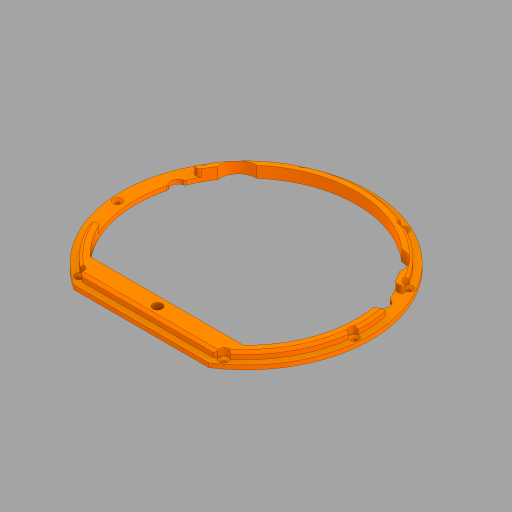
# Autodesk Inventor part: ramka_kriska
Saved by Autodesk Inventor 2024.2 (Build 282272000, 272)
## iProperties
Created: 2024-01-02
Part Number: ramka_kriska
Material: Типовые
Document SubType Name: Modeling
Designer: Fedor Orlov
Density: 1 g/cm^3
Appearance: По умолчанию
Author: Fedor Orlov
Autodesk Inventor part; units mm, degrees
ref_plane "YZ Plane" through (0, 0, 0) normal (1, 0, 0) x (0, 1, 0)
ref_plane "XZ Plane" through (0, 0, 0) normal (0, 1, 0) x (-1, 0, 0)
ref_plane "XY Plane" through (0, 0, 0) normal (0, 0, 1) x (1, 0, 0)
sketch "Эскиз2" plane through (0, 0, 0) normal (0, 1, 0) x (-1, 0, 0)
  circle A0 centre (52.9444, -65.7473) radius 1.5
  circle A1 centre (18.9444, -65.7473) radius 1.5
  circle A2 centre (-32.9359, 24.112) radius 1.5
  circle A3 centre (-15.9359, 53.5568) radius 1.5
  circle A4 centre (87.8247, 53.5568) radius 1.5
  circle A5 centre (104.8247, 24.112) radius 1.5
  arc A6 (-9.0556, 75.9947) -> (-12.1486, 77.6696) centre (-11.0556, 75.9947) ccw construction
  arc A7 (-12.1486, 77.6696) -> (84.0374, 77.6696) centre (35.9444, 3.9738) ccw
  arc A8 (84.0374, 77.6696) -> (80.9444, 75.9947) centre (82.9444, 75.9947) ccw construction
  line L0 (80.9444, 75.9947) -> (80.9444, 72.0979) construction
  arc A9 (78.9444, 70.0979) -> (80.9444, 72.0979) centre (78.9444, 72.0979) ccw construction
  line L1 (78.9444, 70.0979) -> (-7.0556, 70.0979) construction
  arc A10 (-9.0556, 72.0979) -> (-7.0556, 70.0979) centre (-7.0556, 72.0979) ccw construction
  line L2 (-9.0556, 72.0979) -> (-9.0556, 75.9947) construction
  arc A11 (80.2513, 70.5839) -> (-9.0556, 70.1176) centre (35.9444, 3.9738) ccw construction
  line L3 (35.9444, 3.9738) -> (-51.7207, 11.6435) construction
  line L4 (-51.7207, 11.6435) -> (-47.7359, 11.2949) construction
  circle A12 centre (-47.7359, 11.2949) radius 1.5
  line L5 (35.9444, 3.9738) -> (-17.5291, 73.8636) construction
  circle A13 centre (-15.0984, 70.6868) radius 1.5
  line L6 (35.9444, 3.9738) -> (-1.246, -75.7813) construction
  line L7 (35.9444, 3.9738) -> (-40.2658, -40.0262) construction
  circle A14 centre (0.4445, -72.156) radius 1.5
  circle A15 centre (-36.8017, -38.0262) radius 1.5
  line L8 (35.9444, 3.9738) -> (35.9444, -84.0262) construction
  circle A16 centre (86.9873, 70.6868) radius 1.5
  circle A17 centre (119.6248, 11.2949) radius 1.5
  circle A18 centre (108.6906, -38.0262) radius 1.5
  circle A19 centre (71.4444, -72.156) radius 1.5
  line L9 (-7.0556, 70.0979) -> (78.9444, 70.0979) construction
  line L10 (35.9444, 70.0979) -> (35.9444, 66.5979) construction
  circle A20 centre (35.9444, 66.5979) radius 1.5
  line L11 (-19.0246, 62.0979) -> (90.9134, 62.0979)
  arc A21 (80.9444, 70.1176) -> (80.2513, 70.5839) centre (35.9444, 3.9738) ccw construction
  arc A22 (-9.0556, 70.1176) -> (-19.0246, 62.0979) centre (35.9444, 3.9738) ccw construction
  arc A23 (-19.0246, 62.0979) -> (90.9134, 62.0979) centre (35.9444, 3.9738) ccw
  arc A24 (90.9134, 62.0979) -> (80.9444, 70.1176) centre (35.9444, 3.9738) ccw construction
  arc A25 (-11.6466, 77.9947) -> (83.5354, 77.9947) centre (35.9444, 3.9738) ccw
  line L12 (83.5354, 77.9947) -> (-11.6466, 77.9947)
  arc A26 (83.5354, 77.9947) -> (-11.6466, 77.9947) centre (35.9444, 3.9738) ccw construction
  point P0 (0, 0)
  point P1 (60.9444, -70.7473)
  dimension "d30" = 8
  dimension "d55" = 95.182
  constraints: 34 point on circle, 27 centre point, 26 end point, 5 vertical, 4 coincident, 4 horizontal, 4 point on line, 4 symmetric about line, 1 midpoint, 72 other
  measures "d30" distance between parallel lines of L11 L1
  measures "d55" distance of L12.start L12.end
extrude "Выдавливание1" add sketch "Эскиз2" along normal blind 3 contours A25 L12 A7
fillet "Сопряжение1" radius 2 2 edges at (19.0246, 1.5, 62.0979) (-90.9134, 1.5, 62.0979)
sketch "Эскиз3" plane through (0, 3, 0) normal (0, 1, 0) x (1, 0, 0)
  arc A0 (11.6466, -77.9947) -> (-83.5354, -77.9947) centre (-35.9444, -3.9738) ccw projected
  circle A1 centre (-35.9444, -3.9738) radius 84
  arc A2 (11.6466, -77.9947) -> (-83.5354, -77.9947) centre (-35.9444, -3.9738) ccw projected
  line L0 (18.2228, -62.0979) -> (-90.1116, -62.0979) projected
  arc A3 (-91.5006, -61.537) -> (-90.1116, -62.0979) centre (-90.1116, -60.0979) ccw projected
  arc A4 (19.6117, -61.537) -> (-91.5006, -61.537) centre (-35.9444, -3.9738) ccw projected
  arc A5 (18.2228, -62.0979) -> (19.6117, -61.537) centre (18.2228, -60.0979) ccw projected
  circle A6 centre (-86.9873, -70.6868) radius 1.5 projected
  circle A7 centre (47.7359, -11.2949) radius 1.5 projected
  circle A8 centre (36.8017, 38.0262) radius 1.5 projected
  circle A9 centre (-0.4445, 72.156) radius 1.5 projected
  circle A10 centre (-108.6906, 38.0262) radius 1.5 projected
  circle A11 centre (-119.6248, -11.2949) radius 1.5 projected
  circle A12 centre (-71.4444, 72.156) radius 1.5 projected
  circle A13 centre (-35.9444, -66.5979) radius 1.5 projected
  circle A14 centre (15.0984, -70.6868) radius 1.5 projected
  line L1 (-83.5354, -77.9947) -> (11.6466, -77.9947) projected
  line L2 (-82.3456, -73.9947) -> (10.4568, -73.9947)
  point P0 (0, 0)
  point P1 (12.1486, -77.6696)
  point P2 (-84.0374, -77.6696)
  point P3 (-92.4829, -66.0979)
  point P4 (20.5941, -66.0979)
  point P5 (47.5919, -12.788)
  point P6 (47.8533, -9.7995)
  point P7 (37.5401, 36.7205)
  point P8 (36.0401, 39.3185)
  point P9 (0.9093, 71.51)
  point P10 (-1.8096, 72.7778)
  point P11 (-70.0793, 72.7778)
  point P12 (-72.7981, 71.51)
  point P13 (-107.929, 39.3185)
  point P14 (-109.4289, 36.7205)
  point P15 (-119.7422, -9.7995)
  point P16 (-119.4807, -12.788)
  point P17 (13.899, -71.5876)
  point P18 (16.2816, -69.7648)
  point P19 (-88.1704, -69.7648)
  point P20 (-85.7879, -71.5876)
  dimension "d34" = 4
  dimension "d56" = 4
  constraints: 4 point on circle, 2 end point, 1 centre point, 1 coincident, 1 horizontal
  measures "d34" radial gap between concentric circles of A0 A1
  measures "d56" distance between parallel lines of L2 L1
extrude "Выдавливание2" add sketch "Эскиз3" along normal blind 5 contours L2 A1 A6 A11 A10 A12 A9 A8 A7 A14
sketch "Эскиз4" plane through (0, 8, 0) normal (0, 1, 0) x (1, 0, 0)
  arc A0 (16.2816, -69.7648) -> (47.5919, -12.788) centre (-35.9444, -3.9738) ccw projected
  circle A1 centre (-35.9444, -66.5979) radius 1.5 projected
  arc A2 (18.2228, -62.0979) -> (19.6117, -61.537) centre (18.2228, -60.0979) ccw projected
  line L0 (18.2228, -62.0979) -> (-90.1116, -62.0979) projected
  arc A3 (-91.5006, -61.537) -> (-90.1116, -62.0979) centre (-90.1116, -60.0979) ccw projected
  arc A4 (19.6117, -61.537) -> (-91.5006, -61.537) centre (-35.9444, -3.9738) ccw projected
  arc A5 (-90.1116, -60.0979) -> (18.2228, -60.0979) centre (-35.9444, -3.9738) ccw construction
  line L1 (-90.1116, -60.0979) -> (18.2228, -60.0979)
  arc A6 (18.2228, -60.0979) -> (-90.1116, -60.0979) centre (-35.9444, -3.9738) ccw
  arc A7 (10.4568, -73.9947) -> (13.899, -71.5876) centre (-35.9444, -3.9738) ccw projected
  arc A8 (16.2816, -69.7648) -> (13.899, -71.5876) centre (15.0984, -70.6868) ccw projected
  arc A9 (47.8533, -9.7995) -> (47.5919, -12.788) centre (47.7359, -11.2949) ccw projected
  arc A10 (47.8533, -9.7995) -> (37.5401, 36.7205) centre (-35.9444, -3.9738) ccw projected
  arc A11 (36.0401, 39.3185) -> (37.5401, 36.7205) centre (36.8017, 38.0262) ccw projected
  arc A12 (36.0401, 39.3185) -> (0.9093, 71.51) centre (-35.9444, -3.9738) ccw projected
  arc A13 (-1.8096, 72.7778) -> (0.9093, 71.51) centre (-0.4445, 72.156) ccw projected
  arc A14 (-1.8096, 72.7778) -> (-70.0793, 72.7778) centre (-35.9444, -3.9738) ccw projected
  arc A15 (-72.7981, 71.51) -> (-70.0793, 72.7778) centre (-71.4444, 72.156) ccw projected
  arc A16 (-72.7981, 71.51) -> (-107.929, 39.3185) centre (-35.9444, -3.9738) ccw projected
  arc A17 (-109.4289, 36.7205) -> (-107.929, 39.3185) centre (-108.6906, 38.0262) ccw projected
  arc A18 (-109.4289, 36.7205) -> (-119.7422, -9.7995) centre (-35.9444, -3.9738) ccw projected
  arc A19 (-119.4807, -12.788) -> (-119.7422, -9.7995) centre (-119.6248, -11.2949) ccw projected
  arc A20 (-119.4807, -12.788) -> (-88.1704, -69.7648) centre (-35.9444, -3.9738) ccw projected
  arc A21 (-85.7879, -71.5876) -> (-88.1704, -69.7648) centre (-86.9873, -70.6868) ccw projected
  arc A22 (-85.7879, -71.5876) -> (-82.3456, -73.9947) centre (-35.9444, -3.9738) ccw projected
  line L2 (-82.3456, -73.9947) -> (10.4568, -73.9947) projected
  point P0 (0, 0)
  dimension "d38" = 2
  dimension "d39" = 2
  constraints: 4 point on circle, 2 centre point, 2 end point, 1 coincident, 1 horizontal
  measures "d38" radial gap between concentric circles of A4 A5
  measures "d39" distance between parallel lines of L0 L1
extrude "Выдавливание3" add sketch "Эскиз4" against normal blind 8 contours L0 A3 A4 A2
fillet "Сопряжение2" radius 2 2 edges at (18.2228, 4, 60.0979) (-90.1116, 4, 60.0979)
sketch "Эскиз5" plane through (0, 3, 0) normal (0, 1, 0) x (1, 0, 0)
  arc A0 (47.8533, -9.7995) -> (47.5919, -12.788) centre (47.7359, -11.2949) ccw projected
  arc A1 (36.0401, 39.3185) -> (37.5401, 36.7205) centre (36.8017, 38.0262) ccw projected
  arc A2 (-1.8096, 72.7778) -> (0.9093, 71.51) centre (-0.4445, 72.156) ccw projected
  arc A3 (-37.3586, -66.0979) -> (-34.5302, -66.0979) centre (-35.9444, -66.5979) ccw projected
  circle A4 centre (47.7359, -11.2949) radius 3.25
  circle A5 centre (36.8017, 38.0262) radius 3.25
  circle A6 centre (-0.4445, 72.156) radius 3.25
  circle A7 centre (-35.9444, -66.5979) radius 3.25
  circle A8 centre (-71.4444, 72.156) radius 1.5 projected
  circle A9 centre (-71.4444, 72.156) radius 3.25
  arc A10 (-109.4289, 36.7205) -> (-107.929, 39.3185) centre (-108.6906, 38.0262) ccw projected
  circle A11 centre (-108.6906, 38.0262) radius 3.25
  circle A12 centre (-119.6248, -11.2949) radius 1.5 projected
  circle A13 centre (-119.6248, -11.2949) radius 3.25
  circle A14 centre (15.0984, -70.6868) radius 1.5 projected
  circle A15 centre (15.0984, -70.6868) radius 3.25
  circle A16 centre (-86.9873, -70.6868) radius 1.5 projected
  circle A17 centre (-86.9873, -70.6868) radius 3.25
  point P0 (0, 0)
  dimension "d43" = 6.5
  dimension "d44" = 6.5
  dimension "d45" = 6.5
  dimension "d46" = 6.5
  dimension "d47" = 6.5
  dimension "d48" = 6.5
  dimension "d49" = 6.5
  dimension "d57" = 6.5
  dimension "d58" = 6.5
  constraints: 9 centre point, 9 coincident
  measures "d43" diameter of A4
  measures "d44" diameter of A5
  measures "d45" diameter of A6
  measures "d46" diameter of A7
  measures "d47" diameter of A9
  measures "d48" diameter of A11
  measures "d49" diameter of A13
  measures "d57" diameter of A15
  measures "d58" diameter of A17
extrude "Выдавливание4" cut sketch "Эскиз5" along normal blind 8 contours A4 | A5 | A6 | A7 | A8 | A9 | A11 | A12 | A13 | A14 | A15 | A16 | A17
chamfer "Фаска1" distance 1.6 angle 45 9 edges at (49.2359, 3, 11.2949) (38.3017, 3, -38.0262) (1.0555, 3, -72.156) (-69.9444, 3, -72.156) (-107.1906, 3, -38.0262) (-118.1248, 3, 11.2949) (-85.4873, 3, 70.6868) (16.5984, 3, 70.6868) (-34.4444, 3, 66.5979)
sketch "Эскиз6" plane through (0, 8, 0) normal (0, 1, 0) x (1, 0, 0)
  arc A0 (18.813, -59.5222) -> (-90.7019, -59.5222) centre (-35.9444, -3.9738) ccw projected
  arc A1 (9.3615, -73.9947) -> (10.2757, -73.3947) centre (-35.9444, -3.9738) ccw construction
  arc A2 (-74.3627, 70.7258) -> (-107.0114, 40.8088) centre (-35.9444, -3.9738) ccw projected
  line L0 (-82.1645, -73.3947) -> (10.2757, -73.3947)
  line L1 (-82.3456, -73.9947) -> (10.4568, -73.9947) projected
  arc A3 (47.9565, -8.0524) -> (47.3901, -14.5265) centre (47.7359, -11.2949) ccw projected
  arc A4 (47.9565, -8.0524) -> (38.372, 35.1807) centre (-35.9444, -3.9738) ccw projected
  arc A5 (35.1226, 40.8088) -> (38.372, 35.1807) centre (36.8017, 38.0262) ccw projected
  arc A6 (35.1226, 40.8088) -> (2.4739, 70.7258) centre (-35.9444, -3.9738) ccw projected
  arc A7 (-3.416, 73.4723) -> (2.4739, 70.7258) centre (-0.4445, 72.156) ccw projected
  arc A8 (-3.416, 73.4723) -> (-68.4728, 73.4723) centre (-35.9444, -3.9738) ccw projected
  arc A9 (-74.3627, 70.7258) -> (-68.4728, 73.4723) centre (-71.4444, 72.156) ccw projected
  arc A10 (-74.3627, 70.7258) -> (-107.0114, 40.8088) centre (-35.9444, -3.9738) ccw projected
  arc A11 (-110.2608, 35.1807) -> (-107.0114, 40.8088) centre (-108.6906, 38.0262) ccw projected
  arc A12 (-110.2608, 35.1807) -> (-119.8453, -8.0524) centre (-35.9444, -3.9738) ccw projected
  arc A13 (-119.2789, -14.5265) -> (-119.8453, -8.0524) centre (-119.6248, -11.2949) ccw projected
  arc A14 (-119.2789, -14.5265) -> (-89.5298, -68.6624) centre (-35.9444, -3.9738) ccw projected
  arc A15 (-84.3684, -72.6114) -> (-89.5298, -68.6624) centre (-86.9873, -70.6868) ccw projected
  arc A16 (-84.3684, -72.6114) -> (-82.3456, -73.9947) centre (-35.9444, -3.9738) ccw projected
  line L2 (-82.3456, -73.9947) -> (10.4568, -73.9947) projected
  arc A17 (10.4568, -73.9947) -> (12.4796, -72.6114) centre (-35.9444, -3.9738) ccw projected
  arc A18 (17.6409, -68.6624) -> (12.4796, -72.6114) centre (15.0984, -70.6868) ccw projected
  arc A19 (17.6409, -68.6624) -> (47.3901, -14.5265) centre (-35.9444, -3.9738) ccw projected
  circle A20 centre (-35.9444, -66.5979) radius 3.25 projected
  arc A21 (18.813, -59.5222) -> (-90.7019, -59.5222) centre (-35.9444, -3.9738) ccw projected
  arc A22 (17.409, -60.0979) -> (18.813, -59.5222) centre (17.409, -58.0979) ccw projected
  line L3 (17.409, -60.0979) -> (-89.2978, -60.0979) projected
  arc A23 (-90.7019, -59.5222) -> (-89.2978, -60.0979) centre (-89.2978, -58.0979) ccw projected
  arc A24 (-81.2504, -73.9947) -> (9.3615, -73.9947) centre (-35.9444, -3.9738) ccw construction
  arc A25 (-82.1645, -73.3947) -> (-81.2504, -73.9947) centre (-35.9444, -3.9738) ccw construction
  arc A26 (10.2757, -73.3947) -> (-82.1645, -73.3947) centre (-35.9444, -3.9738) ccw
  point P0 (0, 0)
  point P1 (-84.0585, -72.0957)
  point P2 (12.1697, -72.0957)
  point P3 (-89.113, -68.2285)
  point P4 (-118.6892, -14.4073)
  point P5 (-119.2439, -8.0673)
  point P6 (-109.7094, 34.94)
  point P7 (-106.5273, 40.4516)
  point P8 (-74.0491, 70.2124)
  point P9 (-107.0114, 40.8088)
  point P10 (-68.2811, 72.902)
  point P11 (-3.6077, 72.902)
  point P12 (2.1603, 70.2124)
  point P13 (34.6384, 40.4516)
  point P14 (37.8206, 34.94)
  point P15 (47.3551, -8.0673)
  point P16 (46.8004, -14.4073)
  point P17 (17.2242, -68.2285)
  dimension "d59" = 0.6
  dimension "d60" = 0.6
  constraints: 9 point on circle, 4 centre point, 2 end point, 2 point on line, 1 coincident, 1 parallel
  measures "d59" radial gap between concentric circles of A1 A2
  measures "d60" distance between parallel lines of L1 L0
extrude "Выдавливание5" cut sketch "Эскиз6" against normal blind 5 contours A9 A26 A11 A2 | A9 A8 A7 A26 | A26 A13 A12 A11 | A7 A6 A5 A26 | A26 A15 A14 A13 | A5 A4 A3 A26 | A26 L0 A18 A17 L1 A16 A15 | A3 A19 A18 A26
chamfer "Фаска2" distance 1.8 angle 45 8 edges at (37.1466, 8, 44.1393) (45.4787, 8, -14.0772) (20.3998, 8, -57.5151) (-35.9444, 8, -79.4262) (-92.2886, 8, -57.5151) (-117.3675, 8, -14.0772) (-109.0354, 8, 44.1393) (-35.9444, 8, 73.3947)
sketch "Эскиз7" plane through (0, 3, 0) normal (0, 1, 0) x (1, 0, 0)
  circle A0 centre (47.7359, -11.2949) radius 3.1 projected
  line L0 (63.7359, 14.7051) -> (31.7359, 14.7051)
  line L1 (31.7359, 14.7051) -> (31.7359, -37.2949)
  line L2 (31.7359, -37.2949) -> (63.7359, -37.2949)
  line L3 (63.7359, -37.2949) -> (63.7359, 14.7051)
  circle A1 centre (47.7359, -11.2949) radius 1.5 projected
  line L4 (63.7359, 14.7051) -> (31.7359, -37.2949) construction
  line L5 (31.7359, 14.7051) -> (63.7359, -37.2949) construction
  circle A2 centre (-119.6248, -11.2949) radius 1.5 projected
  line L6 (-135.6248, -37.2949) -> (-103.6248, -37.2949)
  line L7 (-103.6248, -37.2949) -> (-103.6248, 14.7051)
  line L8 (-103.6248, 14.7051) -> (-135.6248, 14.7051)
  line L9 (-135.6248, 14.7051) -> (-135.6248, -37.2949)
  line L10 (-135.6248, -37.2949) -> (-103.6248, 14.7051) construction
  line L11 (-103.6248, -37.2949) -> (-135.6248, 14.7051) construction
  point P0 (0, 0)
  dimension "d66" = 32
  dimension "d67" = 52
  dimension "d90" = 32
  dimension "d91" = 52
  constraints: 24 end point, 4 midpoint, 4 parallel, 2 horizontal, 2 perpendicular
  measures "d66" distance of L2.end L1.end
  measures "d67" distance of L1.end L0.end
  measures "d90" distance of L8.end L7.end
  measures "d91" distance of L7.end L6.end
extrude "Выдавливание6" cut sketch "Эскиз7" along normal blind 10 contours A2 | L9 L8 L7 L6
fillet "Сопряжение3" radius 2 4 edges at (-106.4689, 5.5, 37.2949) (-112.3988, 4.6, 37.2949) (-117.2258, 4.6, -14.7051) (-111.6748, 5.5, -14.7051)
sketch "Эскиз8" plane through (0, 0, 0) normal (0, -1, 0) x (1, 0, 0)
  arc A0 (-90.7019, 59.5222) -> (18.813, 59.5222) centre (-35.9444, 3.9738) ccw projected
  arc A1 (-83.5354, 77.9947) -> (11.6466, 77.9947) centre (-35.9444, 3.9738) ccw projected
  line L0 (-120.6085, -20.0262) -> (48.7196, -20.0262) construction
  circle A2 centre (-107.9444, -20.0262) radius 5
  circle A3 centre (36.0556, -20.0262) radius 5
  point P0 (0, 0)
  dimension "d71" = 24
  dimension "d72" = 10
  dimension "d73" = 72
  dimension "d74" = 10
  dimension "d75" = 72
  constraints: 2 centre point, 2 end point, 2 point on circle, 2 point on line, 1 horizontal
  measures "d71" distance from line of L0 A0.centre
  measures "d72" diameter of A2
  measures "d73" horizontal distance of A2.centre A0.centre
  measures "d74" diameter of A3
  measures "d75" horizontal distance of A3.centre A0.centre
extrude "Выдавливание7" cut sketch "Эскиз8" against normal blind 10
sketch "Эскиз9" plane through (0, 3, 0) normal (0, 1, 0) x (1, 0, 0)
  arc A0 (39.3776, 16.2893) -> (36.4711, 25.0089) centre (36.0556, 20.0262) ccw projected
  arc A1 (-108.3599, 25.0089) -> (-111.2664, 16.2893) centre (-107.9444, 20.0262) ccw projected
  circle A2 centre (36.0556, 20.0262) radius 12
  circle A3 centre (-107.9444, 20.0262) radius 12
  point P0 (0, 0)
  dimension "d78" = 24
  dimension "d79" = 24
  constraints: 2 centre point, 2 coincident
  measures "d78" diameter of A2
  measures "d79" diameter of A3
extrude "Выдавливание8" cut sketch "Эскиз9" along normal blind 10
fillet "Сопряжение4" radius 2 2 edges at (39.5293, 4.6, -31.5124) (33.4044, 5.5, -31.7297)
fillet "Сопряжение5" radius 2 2 edges at (-111.4182, 4.6, -31.5124) (-105.2933, 5.5, -31.7297)
fillet "Сопряжение6" radius 2 4 edges at (-111.2664, 1.5, -16.2893) (-108.3599, 1.5, -25.0089) (39.3776, 1.5, -16.2893) (36.4711, 1.5, -25.0089)
sketch "Эскиз10" plane through (0, 3, 0) normal (0, 1, 0) x (1, 0, 0)
  arc A0 (32.74, 32.9918) -> (-104.6288, 32.9918) centre (-35.9444, -3.9738) ccw projected
  line L0 (-35.9444, -3.9738) -> (15.3924, 41.8944)
  line L1 (-35.9444, -3.9738) -> (-35.9444, 108.5274)
  circle A1 centre (15.3924, 41.8944) radius 13
  circle A2 centre (-87.2812, 41.8944) radius 13
  point P0 (0, 0)
  point P1 (-87.1173, 54.8933)
  point P2 (-100.1798, 40.2734)
  dimension "d85" = 68.843
  dimension "d86" = 48.22
  dimension "d87" = 26
  constraints: 4 end point, 2 centre point, 1 coincident, 1 symmetric about line, 1 vertical, 1 other
  measures "d85" distance of L0.start L0.end
  measures "d86" angle of L1 L0
  measures "d87" diameter of A1
extrude "Выдавливание9" cut sketch "Эскиз10" along normal mid plane 20 contours A1 A0 | A0 A1 | A2 A0 | A0 A2
equation "\"d44\" = d43"
equation "\"d75\" = d73"
